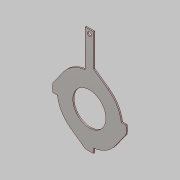
# Autodesk Inventor part: Ground Plate Promag DN50
Saved by Autodesk Inventor 2017 (Build 210142000, 142)
## iProperties
Created: 2018-11-28
Part Number: Ground Plate Promag DN50
Material: 304L
Document SubType Name: Modeling
Designer: Demarec
Density: 8 g/cm^3
Appearance: Semi-Polished
Author: Demarec
Autodesk Inventor part; units mm, degrees
ref_plane "YZ Plane" through (0, 0, 0) normal (1, 0, 0) x (0, 1, 0)
ref_plane "XZ Plane" through (0, 0, 0) normal (0, 1, 0) x (-1, 0, 0)
ref_plane "XY Plane" through (0, 0, 0) normal (0, 0, 1) x (1, 0, 0)
sketch "Sketch1" plane through (0, 0, 0) normal (0, 1, 0) x (-1, 0, 0)
  circle A0 centre (0, 0) radius 26
  circle A1 centre (0, 0) radius 50.5 construction
  line L0 (-6.5, -50.0799) -> (6.5, -50.0799)
  line L1 (6.5, -50.0799) -> (6.5, -108)
  line L2 (6.5, -108) -> (-6.5, -108)
  line L3 (-6.5, -108) -> (-6.5, -50.0799)
  circle A2 centre (0, 0) radius 57.75 construction
  arc A3 (-41.1223, -29.3123) -> (-6.5, -50.0799) centre (0, 0) ccw
  line L4 (-41.1223, -29.3123) -> (-57.383, -6.5)
  arc A4 (-57.383, 6.5) -> (-57.383, -6.5) centre (0, 0) ccw
  line L5 (-57.383, 6.5) -> (-50.0799, 6.5)
  arc A5 (-29.3123, 41.1223) -> (-50.0799, 6.5) centre (0, 0) ccw
  line L6 (-29.3123, 41.1223) -> (-6.5, 57.383)
  arc A6 (6.5, 57.383) -> (-6.5, 57.383) centre (0, 0) ccw
  line L7 (6.5, 57.383) -> (6.5, 50.0799)
  arc A7 (41.1223, 29.3123) -> (6.5, 50.0799) centre (0, 0) ccw
  line L8 (41.1223, 29.3123) -> (57.383, 6.5)
  arc A8 (57.383, -6.5) -> (57.383, 6.5) centre (0, 0) ccw
  line L9 (57.383, -6.5) -> (50.0799, -6.5)
  arc A9 (29.3123, -41.1223) -> (50.0799, -6.5) centre (0, 0) ccw
  line L10 (29.3123, -41.1223) -> (6.5, -57.383)
  circle A10 centre (0, -101.5) radius 3.25
  dimension "DiaB" = 101
  dimension "DiaD" = 115.5
  dimension "DiaA" = 52
  dimension "d2" = 13
  dimension "LenH" = 108
  dimension "d5" = 13
  dimension "d6" = 6.5
  dimension "d7" = 6.5
  dimension "d8" = 13
  dimension "d9" = 6.5
  dimension "d10" = 13
  dimension "d11" = 6.5
  dimension "d12" = 6.5
  dimension "d13" = 6.5
  constraints: 22 end point, 14 point on circle, 9 centre point, 4 tangent, 3 coincident, 3 parallel, 2 horizontal, 1 perpendicular, 1 point on line, 1 vertical, 27 other
  measures "DiaA" diameter of A0
  measures "d2" distance of L1.end L2.end
  measures "LenH" distance from line of L2 point (0, 0)
  measures "d5" distance of L5.start L4.end
  measures "d6" vertical distance of point (0, 0) L4.end
  measures "d7" horizontal distance of L6.end A3.centre
  measures "d8" distance of L7.start L6.end
  measures "d9" vertical distance of A8.centre L8.end
  measures "d10" distance of L9.start L8.end
  measures "d11" diameter of A10
  measures "d12" distance from line of A10.centre L2
  measures "d13" distance from line of A10.centre L3
extrude "Extrusion1" add sketch "Sketch1" along normal blind 2
equation "\"d5\" = d2"
equation "\"d6\" = 0.5 * d2"
equation "\"d7\" = d6"
equation "\"d8\" = d5"
equation "\"d9\" = d6"
equation "\"d10\" = d5"
equation "\"d12\" = 0.5 * d2"
equation "\"d13\" = 0.5 * d2"
body "Solid1"
